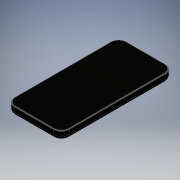
# Autodesk Inventor part: Andoid Phone
Saved by Autodesk Inventor 2016 (Build 200138000, 138)
## iProperties
Created: 2015-09-05
Part Number: Andoid Phone
Material: ABS Plastic
Document SubType Name: Modeling
Designer: Tim
Density: 1.06 g/cm^3
Appearance: Black
Author: Tim
Autodesk Inventor part; units mm, degrees
ref_plane "YZ Plane" through (0, 0, 0) normal (1, 0, 0) x (0, 1, 0)
ref_plane "XZ Plane" through (0, 0, 0) normal (0, 1, 0) x (-1, 0, 0)
ref_plane "XY Plane" through (0, 0, 0) normal (0, 0, 1) x (1, 0, 0)
sketch "Sketch1" plane through (0, 0, 0) normal (0, 0, 1) x (1, 0, 0)
  line L0 (33.02, -67.31) -> (-33.02, -67.31)
  line L1 (-33.02, -67.31) -> (-33.02, 67.31)
  line L2 (-33.02, 67.31) -> (33.02, 67.31)
  line L3 (33.02, 67.31) -> (33.02, -67.31)
  line L4 (33.02, -67.31) -> (-33.02, 67.31) construction
  line L5 (-33.02, -67.31) -> (33.02, 67.31) construction
  point P0 (0, 0)
  dimension "d0" = 66.04
  dimension "d1" = 134.62
  constraints: 12 end point, 2 midpoint, 2 parallel, 1 horizontal, 1 perpendicular
  measures "d0" distance of L1.end L2.end
  measures "d1" distance of L0.end L1.end
extrude "Extrusion1" add sketch "Sketch1" along normal blind 10.16
fillet "Fillet1" radius 10 4 edges at (33.02, 67.31, 5.08) (-33.02, 67.31, 5.08) (33.02, -67.31, 5.08) (-33.02, -67.31, 5.08)
fillet "Fillet2" radius 4 8 edges at (30.0911, -64.3811, 0) (0, -67.31, 0) (-30.0911, -64.3811, 0) (-33.02, 0, 0) (-30.0911, 64.3811, 0) (0, 67.31, 0) (30.0911, 64.3811, 0) (33.02, 0, 0)
fillet "Fillet3" radius 1 8 edges at (30.0911, 64.3811, 10.16) (0, 67.31, 10.16) (-30.0911, 64.3811, 10.16) (-33.02, 0, 10.16) (-30.0911, -64.3811, 10.16) (0, -67.31, 10.16) (30.0911, -64.3811, 10.16) (33.02, 0, 10.16)
body "Solid1"
